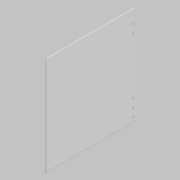
# Autodesk Inventor part: Front
Saved by Autodesk Inventor 2020 (Build 240168000, 168)
## iProperties
Created: 2020-08-05
Part Number: Front
Material: Generic
Document SubType Name: Modeling
Designer: Abbas
Density: 1 g/cm^3
Appearance: Default
Author: Abbas
Autodesk Inventor part; units mm, degrees
ref_plane "YZ Plane" through (0, 0, 0) normal (1, 0, 0) x (0, 1, 0)
ref_plane "XZ Plane" through (0, 0, 0) normal (0, 1, 0) x (-1, 0, 0)
ref_plane "XY Plane" through (0, 0, 0) normal (0, 0, 1) x (1, 0, 0)
sketch "Sketch1" plane through (0, 0, 0) normal (1, 0, 0) x (0, 1, 0)
  line L0 (156, 140) -> (-156, 140)
  line L1 (-156, 140) -> (-156, -140)
  line L2 (-156, -140) -> (156, -140)
  line L3 (156, -140) -> (156, 140)
  line L4 (156, 140) -> (-156, -140) construction
  line L5 (-156, 140) -> (156, -140) construction
  circle A0 centre (140.989, -134.477) radius 1.875
  circle A1 centre (115.189, -134.477) radius 1.875
  circle A2 centre (89.389, -134.477) radius 1.875
  line L6 (0, 0) -> (0, -46.8425)
  circle A3 centre (-140.989, -134.477) radius 1.875
  circle A4 centre (-115.189, -134.477) radius 1.875
  circle A5 centre (-89.389, -134.477) radius 1.875
  dimension "d0" = 312
  dimension "d1" = 280
  dimension "d2" = 3.75
  dimension "d3" = 3.75
  dimension "d4" = 15.011
  dimension "d5" = 3.75
  dimension "d6" = 25.8
  dimension "d7" = 25.8
  dimension "d8" = 5.523
  constraints: 14 end point, 6 centre point, 3 symmetric about line, 2 midpoint, 2 parallel, 1 horizontal, 1 perpendicular, 1 vertical, 3 other
  measures "d0" distance of L2.end L1.end
  measures "d1" distance of L1.end L0.end
  measures "d2" diameter of A0
  measures "d3" diameter of A1
  measures "d4" distance from line of L3 A0.centre
  measures "d5" diameter of A2
  measures "d6" distance of A1.centre A0.centre
  measures "d7" distance of A1.centre A2.centre
  measures "d8" distance from line of L2 A0.centre
extrude "Extrusion1" add sketch "Sketch1" along normal blind 3
body "Solid1"
